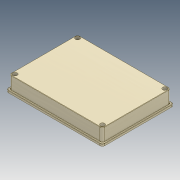
# Autodesk Inventor part: caixa-gabinete-tampa
Saved by Autodesk Inventor 2017 (Build 210142000, 142)
## iProperties
Created: 2018-08-05
Part Number: caixa-gabinete-tampa
Material: ABS Plastic
Document SubType Name: Modeling
Designer: Luiz Gustavo
Density: 1.06 g/cm^3
Appearance: Light Beige
Author: Luiz Gustavo
Autodesk Inventor part; units mm, degrees
ref_plane "YZ Plane" through (0, 0, 0) normal (1, 0, 0) x (0, 1, 0)
ref_plane "XZ Plane" through (0, 0, 0) normal (0, 1, 0) x (-1, 0, 0)
ref_plane "XY Plane" through (0, 0, 0) normal (0, 0, 1) x (1, 0, 0)
sketch "Sketch1" plane through (0, 0, 0) normal (0, 0, 1) x (1, 0, 0)
  line L0 (-150, 110) -> (150, 110)
  line L1 (150, 110) -> (150, -110)
  line L2 (150, -110) -> (-150, -110)
  line L3 (-150, -110) -> (-150, 110)
  line L4 (-150, 110) -> (150, -110) construction
  line L5 (150, 110) -> (-150, -110) construction
  point P0 (0, 0)
  dimension "d0" = 300
  dimension "d1" = 220
  constraints: 12 end point, 2 midpoint, 2 parallel, 1 horizontal, 1 perpendicular
  measures "d0" distance of L1.end L2.end
  measures "d1" distance of L0.end L1.end
extrude "Extrusion1" add sketch "Sketch1" along normal blind 48
sketch "Sketch2" plane through (0, 0, 0) normal (0, 0, 1) x (1, 0, 0)
  line L0 (-155, -115) -> (155, -115)
  line L1 (155, -115) -> (155, 115)
  line L2 (155, 115) -> (-155, 115)
  line L3 (-155, 115) -> (-155, -115)
  line L4 (-155, -115) -> (155, 115) construction
  line L5 (155, -115) -> (-155, 115) construction
  point P0 (0, 0)
  dimension "d4" = 310
  dimension "d5" = 230
  constraints: 12 end point, 2 midpoint, 2 parallel, 1 horizontal, 1 perpendicular
  measures "d4" distance of L2.end L1.end
  measures "d5" distance of L1.end L0.end
extrude "Extrusion2" add sketch "Sketch2" along normal blind 7
fillet "Fillet1" radius 8 8 edges at (-150, -110, 27.5) (-155, -115, 3.5) (155, -115, 3.5) (150, -110, 27.5) (155, 115, 3.5) (150, 110, 27.5) (-155, 115, 3.5) (-150, 110, 27.5)
fillet "Fillet2" radius 1 24 edges at (152.6569, -112.6569, 7) (155, 0, 7) (152.6569, 112.6569, 7) (0, 115, 7) (-152.6569, 112.6569, 7) (-155, 0, 7) (-152.6569, -112.6569, 7) (0, -115, 7) (147.6569, -107.6569, 7) (150, 0, 7) (147.6569, 107.6569, 7) (0, 110, 7) (-147.6569, 107.6569, 7) (-150, 0, 7) (-147.6569, -107.6569, 7) (0, -110, 7) (147.6569, -107.6569, 48) (150, 0, 48) (147.6569, 107.6569, 48) (0, 110, 48) (-147.6569, 107.6569, 48) (-150, 0, 48) (-147.6569, -107.6569, 48) (0, -110, 48)
sketch "Sketch3" plane through (0, 0, 0) normal (0, 0, 1) x (1, 0, 0)
  line L0 (-147.5, 107.5) -> (-126.5, 107.5) construction
  line L1 (147.5, 107.5) -> (147.5, 86.5) construction
  line L2 (147.5, -107.5) -> (126.5, -107.5) construction
  line L3 (-147.5, -107.5) -> (-147.5, -86.5) construction
  line L4 (-147.5, 107.5) -> (147.5, -107.5) construction
  line L5 (147.5, 107.5) -> (-147.5, -107.5) construction
  line L6 (-140.5, 100.5) -> (140.5, 100.5) construction
  line L7 (140.5, 100.5) -> (140.5, -100.5) construction
  line L8 (140.5, -100.5) -> (-140.5, -100.5) construction
  line L9 (-140.5, -100.5) -> (-140.5, 100.5) construction
  line L10 (-140.5, 100.5) -> (140.5, -100.5) construction
  line L11 (140.5, 100.5) -> (-140.5, -100.5) construction
  circle A0 centre (-140.5, -100.5) radius 14
  circle A1 centre (140.5, -100.5) radius 14
  circle A2 centre (140.5, 100.5) radius 14
  circle A3 centre (-140.5, 100.5) radius 14
  line L12 (-140.5, -86.5) -> (-147.5, -86.5)
  line L13 (-126.5, -100.5) -> (-126.5, -107.5)
  line L14 (126.5, -100.5) -> (126.5, -107.5)
  line L15 (140.5, -86.5) -> (147.5, -86.5)
  line L16 (-126.5, 100.5) -> (-126.5, 107.5)
  line L17 (-140.5, 86.5) -> (-147.5, 86.5)
  line L18 (126.5, 100.5) -> (126.5, 107.5)
  line L19 (140.5, 86.5) -> (147.5, 86.5)
  line L20 (-147.5, -86.5) -> (-147.5, 86.5)
  line L21 (-126.5, -107.5) -> (-147.5, -107.5) construction
  line L22 (126.5, -107.5) -> (-126.5, -107.5)
  line L23 (147.5, -86.5) -> (147.5, -107.5) construction
  line L24 (147.5, 86.5) -> (147.5, -86.5)
  line L25 (126.5, 107.5) -> (147.5, 107.5) construction
  line L26 (-126.5, 107.5) -> (126.5, 107.5)
  line L27 (-147.5, 86.5) -> (-147.5, 107.5) construction
  point P0 (0, 0)
  point P1 (0, 0)
  point P2 (0, 0)
  dimension "d10" = 295
  dimension "d11" = 215
  dimension "d16" = 281
  dimension "d17" = 201
  dimension "d18" = 28
  constraints: 56 end point, 28 perpendicular, 20 parallel, 11 point on line, 8 point on circle, 6 midpoint, 6 tangent, 4 centre point, 4 coincident, 4 horizontal, 3 equal radius
  measures "d10" distance of L2.start L3.start
  measures "d11" distance of L1.start L2.start
  measures "d16" distance of L7.end L8.end
  measures "d17" distance of L6.end L7.end
  measures "d18" diameter of A0
extrude "Extrusion3" cut sketch "Sketch3" along normal blind 45 contours A0 L12 L20 L17 A3 L16 L26 L18 A2 L19 L24 L15 A1 L14 L22 L13
hole "Hole1" at (-140.5, -100.5, 0) direction (0, 0, 1) diameter 14 end through all
hole "Hole2" at (140.5, -100.5, 0) direction (0, 0, 1) diameter 14 end through all
hole "Hole3" at (-140.5, 100.5, 0) direction (0, 0, 1) diameter 14 end through all
hole "Hole4" at (140.5, 100.5, 0) direction (0, 0, 1) diameter 14 end through all
sketch "Sketch4" plane through (0, 0, 0) normal (0, 0, 1) x (1, 0, 0)
  line L0 (-125, -107.5) -> (-102, -107.5)
  line L1 (-102, -107.5) -> (-102, -102.5)
  line L2 (-102, -102.5) -> (-125, -102.5)
  line L3 (-125, -102.5) -> (-125, -107.5)
  line L4 (-126.5, -107.5) -> (126.5, -107.5) projected
  line L5 (0, -107.5) -> (0, 0) construction
  line L6 (125, -107.5) -> (102, -107.5)
  line L7 (102, -107.5) -> (102, -102.5)
  line L8 (102, -102.5) -> (125, -102.5)
  line L9 (125, -102.5) -> (125, -107.5)
  dimension "d57" = 23
  dimension "d58" = 5
  dimension "d59" = 204
  constraints: 18 end point, 4 symmetric about line, 2 parallel, 1 horizontal, 1 midpoint, 1 perpendicular, 1 point on line, 1 vertical
  measures "d57" distance of L1.end L2.end
  measures "d58" distance of L0.end L1.end
  measures "d59" distance between parallel lines of L1 L7
extrude "Extrusion4" add sketch "Sketch4" along normal up to next
body "Solid1"
